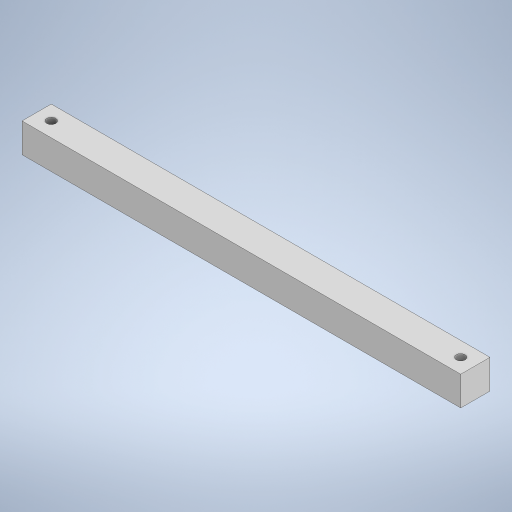
# Autodesk Inventor part: Shita
Saved by Autodesk Inventor 2023 (Build 270158000, 158)
## iProperties
Created: 2022-10-26
Part Number: Shita
Material: 一般
Document SubType Name: Modeling
Designer: banru
Density: 1 g/cm^3
Appearance: 既定
Author: banru
Autodesk Inventor part; units mm, degrees
ref_plane "YZ Plane" through (0, 0, 0) normal (1, 0, 0) x (0, 1, 0)
ref_plane "XZ Plane" through (0, 0, 0) normal (0, 1, 0) x (-1, 0, 0)
ref_plane "XY Plane" through (0, 0, 0) normal (0, 0, 1) x (1, 0, 0)
sketch "スケッチ1" plane through (0, 0, 0) normal (0, 1, 0) x (-1, 0, 0)
  line L0 (0, 0) -> (150, 0)
  line L1 (150, 0) -> (150, -10)
  line L2 (150, -10) -> (0, -10)
  line L3 (0, -10) -> (0, 0)
  dimension "d0" = 150
  dimension "d1" = 10
  constraints: 8 end point, 2 parallel, 1 horizontal, 1 perpendicular
  measures "d0" distance of L1.end L2.end
  measures "d1" distance of L0.end L1.end
extrude "押し出し1" add sketch "スケッチ1" along normal blind 10
sketch "スケッチ2" plane through (0, 10, 0) normal (0, 1, 0) x (1, 0, 0)
  line L0 (-150, 10) -> (-150, 0) projected
  line L1 (0, 0) -> (0, 10) projected
  point P0 (-5, 5)
  point P1 (-145, 5)
  point P2 (-150, 5)
  point P3 (0, 5)
  point P4 (0, 5)
  point P5 (-150, 5)
  dimension "d4" = 5
  dimension "d5" = 5
  constraints: 4 midpoint, 2 horizontal alignment
  measures "d4" distance of point (0, 5) point (-5, 5)
  measures "d5" distance of point (-150, 5) point (-145, 5)
hole "穴1" at (-5, 10, -5) at (-145, 10, -5) direction (0, -1, 0) diameter 3.1 end through all
